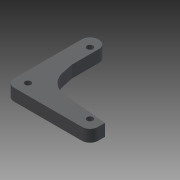
# Autodesk Inventor part: xMotorSpacer
Saved by Autodesk Inventor 2013 (Build 170138000, 138)
## iProperties
Created: 2015-01-14
Part Number: xMotorSpacer
Material: Generic
Document SubType Name: Modeling
Designer: dzban
Density: 1 g/cm^3
Author: dzban
Autodesk Inventor part; units mm, degrees
ref_plane "YZ Plane" through (0, 0, 0) normal (1, 0, 0) x (0, 1, 0)
ref_plane "XZ Plane" through (0, 0, 0) normal (0, 1, 0) x (-1, 0, 0)
ref_plane "XY Plane" through (0, 0, 0) normal (0, 0, 1) x (1, 0, 0)
sketch "Sketch1" plane through (0, 0, 0) normal (0, 0, 1) x (1, 0, 0)
  line L0 (21, -13.5) -> (0, -11.5)
  arc A0 (-11.249, -2.3894) -> (0, -11.5) centre (0, 0) ccw
  line L1 (-11.249, -2.3894) -> (-12.5, 3.5)
  line L2 (-12.5, 3.5) -> (-12.5, 17)
  arc A1 (-12.5, 17) -> (-16.5, 21) centre (-16.5, 17) ccw
  line L3 (-16.5, 21) -> (-17, 21)
  arc A2 (-17, 21) -> (-21, 17) centre (-17, 17) ccw
  line L4 (-21, 17) -> (-21, -17)
  arc A3 (-21, -17) -> (-17, -21) centre (-17, -17) ccw
  line L5 (-17, -21) -> (17, -21)
  arc A4 (17, -21) -> (21, -17) centre (17, -17) ccw
  line L6 (21, -17) -> (21, -13.5)
  circle A5 centre (15.5, -15.5) radius 1.5
  circle A6 centre (-15.5, -15.5) radius 1.5
  circle A7 centre (-15.5, 15.5) radius 1.5
  constraints: 14 end point, 10 point on circle, 8 centre point
extrude "Extrusion1" add sketch "Sketch1" along normal blind 6
body "Solid1"
